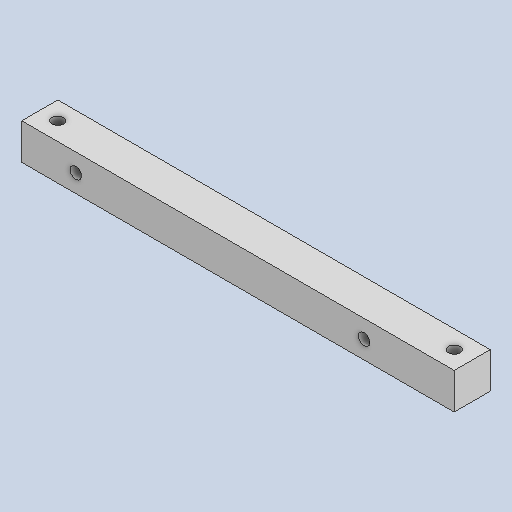
# Autodesk Inventor part: kaku_1010_onetire_plate
Saved by Autodesk Inventor 2025.1 (Build 291241000, 241)
## iProperties
Created: 2024-11-12
Part Number: kaku_1010_onetire_plate
Material: 一般
Document SubType Name: Modeling
Designer: yuki0520
Density: 1 g/cm^3
Appearance: 既定
Author: yuki0520
Autodesk Inventor part; units mm, degrees
ref_plane "YZ Plane" through (0, 0, 0) normal (1, 0, 0) x (0, 1, 0)
ref_plane "XZ Plane" through (0, 0, 0) normal (0, 1, 0) x (-1, 0, 0)
ref_plane "XY Plane" through (0, 0, 0) normal (0, 0, 1) x (1, 0, 0)
derived "zzz_yoko3.ipt"
sketch "スケッチ1" plane through (0, 0, 0) normal (0, 0, 1) x (1, 0, 0)
  circle A0 centre (0, 0) radius 77
  line L0 (45, -80) -> (-45, -80)
  line L1 (-45, -80) -> (-45, 80)
  line L2 (-45, 80) -> (45, 80)
  line L3 (45, 80) -> (45, -80)
  line L4 (45, -80) -> (-45, 80) construction
  line L5 (-45, -80) -> (45, 80) construction
  circle A1 centre (197, 0) radius 120
  circle A2 centre (0, 197) radius 120
  line L6 (-45, 0) -> (45, 0)
  arc A3 (317, 0) -> (0, 317) centre (0, 0) ccw
  line L7 (0, 0) -> (0, 317) construction
  line L8 (0, 0) -> (317, 0) construction
  line L9 (0, 317) -> (0, 0)
  line L10 (317, 0) -> (0, 0)
  line L11 (335.5, -103) -> (317, -103)
  line L12 (317, -103) -> (317, 103)
  line L13 (317, 103) -> (335.5, 103)
  line L14 (335.5, 103) -> (335.5, -103)
  line L15 (335.5, -103) -> (317, 103) construction
  line L16 (317, -103) -> (335.5, 103) construction
  line L17 (-103, 317) -> (-103, 335.5)
  line L18 (-103, 335.5) -> (103, 335.5)
  line L19 (103, 335.5) -> (103, 317)
  line L20 (103, 317) -> (-103, 317)
  line L21 (-35, -80) -> (-35, 345.5)
  line L22 (0, 317) -> (0, 347)
  line L23 (317, 0) -> (347, 0)
  line L24 (227.3, -103) -> (166.7, -103)
  line L25 (166.7, -103) -> (166.7, 103)
  line L26 (166.7, 103) -> (227.3, 103)
  line L27 (227.3, 103) -> (227.3, -103)
  line L28 (227.3, -103) -> (166.7, 103) construction
  line L29 (166.7, -103) -> (227.3, 103) construction
  line L30 (197, 103) -> (197, -103)
  line L31 (-45, 94) -> (355, 94)
  line L32 (-45, -94) -> (355, -94)
  line L33 (35, -80) -> (35, 345.5)
  line L34 (-113, 335.5) -> (113, 335.5)
  line L35 (113, 335.5) -> (113, 345.5)
  line L36 (113, 345.5) -> (-113, 345.5)
  line L37 (-113, 345.5) -> (-113, 335.5)
  line L38 (35, 345.5) -> (45, 345.5)
  line L39 (45, 345.5) -> (45, 355.5)
  line L40 (45, 355.5) -> (35, 355.5)
  line L41 (35, 355.5) -> (35, 345.5)
  circle A4 centre (0, 0) radius 9
  line L42 (335.5, 113) -> (345.5, 113)
  line L43 (345.5, 113) -> (345.5, -107)
  line L44 (345.5, -107) -> (335.5, -107)
  line L45 (335.5, -107) -> (335.5, 113)
  arc A5 (345.5, 113) -> (113, 345.5) centre (0, 0) ccw
  line L46 (103, 335.5) -> (103, 299.7999)
  line L47 (335.5, 103) -> (299.7999, 103)
  line L48 (113, 345.5) -> (113, 296.1756)
  line L49 (-40, -80) -> (-30, -80)
  line L50 (-30, -80) -> (-30, 355.5)
  line L51 (-30, 355.5) -> (-40, 355.5)
  line L52 (-40, 345.5) -> (-40, -80)
  line L53 (-45, -75) -> (345.5, -75)
  line L54 (345.5, -75) -> (345.5, -65)
  line L55 (345.5, -65) -> (-45, -65)
  line L56 (-45, -65) -> (-45, -75)
  line L57 (-40, 345.5) -> (-50, 345.5)
  line L58 (-30, 355.5) -> (-40, 355.5)
  line L59 (-50, 345.5) -> (-40, 345.5)
  line L60 (-40, 345.5) -> (-40, 355.5)
  line L61 (-40, 355.5) -> (-50, 355.5)
  line L62 (-50, 355.5) -> (-50, 345.5)
  line L63 (-45, 80) -> (-55, 80)
  line L64 (-55, 80) -> (-55, 70)
  line L65 (-55, 70) -> (-45, 70)
  line L66 (-45, 70) -> (-45, 80)
  line L67 (-45, -80) -> (-55, -80)
  line L68 (75, -65) -> (75, -75)
  line L69 (-45, -80) -> (345.5, -80)
  line L70 (-45, -65) -> (-70, -65)
  line L71 (-70, -65) -> (-70, -75)
  line L72 (-70, -75) -> (-45, -75)
  line L73 (-45, -75) -> (-45, -65)
  line L74 (345.5, -75) -> (370.5, -75)
  line L75 (370.5, -75) -> (370.5, -65)
  line L76 (370.5, -65) -> (345.5, -65)
  line L77 (345.5, -65) -> (345.5, -75)
  line L78 (-103, 335.5) -> (-103, 345.5)
  point P0 (326.25, 0)
  point P1 (0, 335.5)
  point P2 (197, 0)
  point P3 (-40, 80)
  point P4 (-30, 80)
  point P5 (45, -75)
  point P6 (45, -65)
extrude "押し出し1" add sketch "スケッチ1" along normal blind 10 contours L55 L3 L53 L33 A0 | A0 L33 L55 | L55 L68 L53 L3 | L33 L53 A0 | A0 L53 L50 L55 L33 | L50 A0 L21 L55 | L53 L50 A0 | L50 L53 L21 A0 | L21 A0 L52 L55 | L21 L53 L52 A0 | L52 A0 L55 | L52 L53 L1 L55 A0
sketch "スケッチ4" plane through (-45, -75, 10) normal (0, 0, 1) x (1, 0, 0)
  line L0 (120, 0) -> (120, 10) projected
  line L1 (120, 5) -> (10, 5)
  line L2 (0, 10) -> (0, 0) projected
  point P0 (45, 75)
  point P1 (95, 5)
  point P2 (15, 5)
  point P3 (0, 0)
  dimension "d21" = 25
  dimension "d22" = 15
  constraints: 2 end point, 2 point on line, 1 horizontal, 1 midpoint, 1 other
  measures "d21" distance from line of L0 point (95, 5)
hole "穴3" at (50, -70, 10) at (-30, -70, 10) direction (0, 0, -1) diameter 3.2 end through all
sketch "スケッチ5" plane through (-45, -65, 0) normal (0, 1, 0) x (1, 0, 0)
  line L0 (120, 0) -> (120, -10) projected
  line L1 (120, -5) -> (0, -5)
  line L2 (0, 0) -> (0, -10) projected
  point P0 (45, 0)
  point P1 (115, -5)
  point P2 (5, -5)
  dimension "d30" = 5
  dimension "d31" = 5
  constraints: 2 end point, 2 midpoint, 2 point on line
  measures "d30" distance from line of L0 point (115, -5)
  measures "d31" distance from line of L2 point (5, -5)
hole "穴4" at (70, -65, 5) at (-40, -65, 5) direction (0, -1, 0) diameter 3.2 end through all
